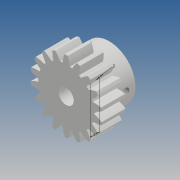
# Autodesk Inventor part: polea aluminio
Saved by Autodesk Inventor 2017 (Build 210142000, 142)
## iProperties
Part Number: polea aluminio
Material: Genérico
Document SubType Name: Modeling
Designer: Leo
Density: 1 g/cm^3
Appearance: Valor por defecto
Author: Leo
Autodesk Inventor part; units mm, degrees
ref_plane "YZ Plane" through (0, 0, 0) normal (1, 0, 0) x (0, 1, 0)
ref_plane "XZ Plane" through (0, 0, 0) normal (0, 1, 0) x (-1, 0, 0)
ref_plane "XY Plane" through (0, 0, 0) normal (0, 0, 1) x (1, 0, 0)
sketch "Boceto1" plane through (0, 0, 0) normal (0, 1, 0) x (-1, 0, 0)
  circle A0 centre (0, 0) radius 3.15
  circle A1 centre (0, 0) radius 11
  line L0 (-5.0187, 2.75) -> (-8.0187, 2.75)
  line L1 (-8.0187, 2.75) -> (-8.0187, -2.75)
  line L2 (-8.0187, -2.75) -> (-5.0187, -2.75)
  line L3 (-5.0187, -2.75) -> (-5.0187, 2.75)
  circle A2 centre (0, 0) radius 7.075 construction
  line L4 (4.8909, -2.9713) -> (0.1278, -5.7213)
  line L5 (6.3909, -5.5694) -> (4.8909, -2.9713)
  line L6 (1.6278, -8.3194) -> (6.3909, -5.5694)
  line L7 (0.1278, -5.7213) -> (1.6278, -8.3194)
  line L8 (0.1278, 5.7213) -> (4.8909, 2.9713)
  line L9 (1.6278, 8.3194) -> (0.1278, 5.7213)
  line L10 (6.3909, 5.5694) -> (1.6278, 8.3194)
  line L11 (4.8909, 2.9713) -> (6.3909, 5.5694)
  point P0 (-5.0187, 0)
  point P1 (-6.5187, 2.75)
  point P2 (2.5093, -4.3463)
  point P3 (0.8778, -7.0203)
  point P4 (2.5093, 4.3463)
  point P5 (5.6409, 4.2703)
  dimension "d0" = 6.3
  dimension "tuerca" = 5.5
  dimension "d2" = 7.85
  dimension "d3" = 3.925
  dimension "d4" = 3
  dimension "d18" = 360
  dimension "d27" = 22
  constraints: 24 end point, 2 centre point, 2 coincident, 2 midpoint, 2 parallel, 1 horizontal, 1 horizontal alignment, 1 perpendicular, 34 other
  measures "d0" diameter of A0
  measures "tuerca" distance of L0.end L1.end
  measures "d2" radial gap between concentric circles of A1 A0
  measures "d4" distance of L0.start L0.end
  measures "d27" diameter of A1
extrude "Extrusión1" add sketch "Boceto1" along normal blind 8 contours A1 | L3 L2 L1 L0 | L5 L6 L7 L4 | L9 L10 L11 L8
sketch "Boceto2" plane through (0, 0, 0) normal (1, 0, 0) x (0, 1, 0)
  circle A0 centre (4, 0) radius 1.5
  point P0 (0, 0)
  dimension "d7" = 3
  dimension "d26" = 4
  constraints: 1 centre point, 1 horizontal alignment
  measures "d7" diameter of A0
  measures "d26" distance of A0.centre point (0, 0)
extrude "Extrusión2" cut sketch "Boceto2" along normal blind 20
sketch "Boceto3" plane through (0, 0, 0) normal (0, -1, 0) x (1, 0, 0)
  circle A0 centre (0, 0) radius 3.15 projected
  circle A1 centre (0, 0) radius 17.939
  constraints: 1 centre point
extrude "Extrusión4" add sketch "Boceto3" along normal blind 10
spur gear teeth "iFeature1:3" teeth 18 pitch diameter 27 tip diameter 30 root diameter 23.25 face width 10 trims to tip circle yes start plane through (0, 0, 0) normal (0, 1, 0) x (-1, 0, 0)
thread "Rosca1" size "M3x0.5" class "6H" standard "ANSI Metric M Profile" full length
pattern_circular "Patrón circular2" count 3 over 360 about axis through (0, -10, 0) along (0, 1, 0) of "Extrusión2"
equation "\"d3\" = 0.5 * d2"
